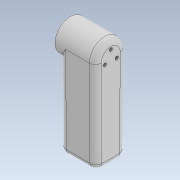
# Autodesk Inventor part: shank_link
Saved by Autodesk Inventor 2020 (Build 240168000, 168)
## iProperties
Created: 2020-12-22
Part Number: shank_link
Material: Generic
Document SubType Name: Modeling
Designer: DELL
Density: 1 g/cm^3
Appearance: Default
Author: DELL
Autodesk Inventor part; units mm, degrees
ref_plane "XY Plane" through (0, 0, 0) normal (0, 0, 1) x (1, 0, 0)
sketch "Sketch1" plane through (0, 0, 0) normal (1, 0, 0) x (0, 1, 0)
  line L0 (0, 0) -> (0, 25.2399) construction
  line L1 (0, 0) -> (0, -46.7601) construction
  line L2 (0, 0) -> (-156, 0) construction
  circle A0 centre (0, 0) radius 26
  line L3 (0, 0) -> (-13, 22.5167) construction
  line L4 (0, 0) -> (-13, -22.5167) construction
  line L5 (-0.1668, 25.9995) -> (-156, 25)
  line L6 (-0.1668, -25.9995) -> (-156, -25)
  line L7 (-156, 25) -> (-156, -25)
  circle A1 centre (0, 0) radius 11.5 construction
  circle A2 centre (11.5, 0) radius 1.65
  line L8 (0, 0) -> (26, 0) construction
  circle A3 centre (-5.75, 9.9593) radius 1.65
  circle A4 centre (-5.75, -9.9593) radius 1.65
  circle A5 centre (0, 0) radius 9.715 construction
  line L9 (0, 0) -> (5.75, 9.9593) construction
  line L10 (0, 0) -> (5.75, -9.9593) construction
  circle A6 centre (4.8575, 8.4134) radius 2
  circle A7 centre (4.8575, -8.4134) radius 2
  circle A8 centre (-9.715, 0) radius 2
  circle A9 centre (11.5, 0) radius 2.75
  circle A10 centre (-5.75, -9.9593) radius 2.75
  circle A11 centre (-5.75, 9.9593) radius 2.75
  circle A12 centre (0, 0) radius 156 construction
  arc A13 (-153.9817, 25.0129) -> (-153.9817, -25.0129) centre (0, 0) ccw
  line L11 (0, 0) -> (-0.1668, 25.9995) construction
  point P0 (-78, 0)
  dimension "d6" = 52
  dimension "d8" = 60
  dimension "d84" = 156
  dimension "d85" = 50
  dimension "d97" = 23
  dimension "d98" = 3.3
  dimension "d99" = 19.43
  dimension "d100" = 30
  dimension "d101" = 4
  dimension "d102" = 5.5
  dimension "d129" = 25.0129
  dimension "d130" = 153.9817
  dimension "d131" = 2.0183
  constraints: 24 end point, 18 point on circle, 14 centre point, 10 point on line, 7 coincident, 6 equal radius, 2 midpoint, 2 vertical, 1 horizontal, 1 perpendicular, 1 symmetric about line, 1 tangent, 3 other
  measures "d6" diameter of A0
  measures "d8" angle of L2 L3
  measures "d84" distance between parallel lines of L7 L1
  measures "d85" distance of L5.end L6.end
  measures "d97" diameter of A1
  measures "d98" diameter of A2
  measures "d99" diameter of A5
  measures "d100" angle of L0 L9
  measures "d101" diameter of A6
  measures "d102" diameter of A9
  measures "d129" distance from line of A12.end L2
  measures "d130" distance from line of L0 A12.end
  measures "d131" distance from line of L7 A12.end
ref_plane "Work Plane1" through (14.5, 0, 0) normal (1, 0, 0) x (0, 1, 0)
ref_plane "Work Plane2" through (20, 0, 0) normal (1, 0, 0) x (0, 1, 0)
extrude "Extrusion4" add sketch "Sketch1" along normal mid plane 70 contours A0 | A6 | A7 | A8 | A9 | A10 | A11
extrude "Extrusion6" cut sketch "Sketch1" against normal blind 40 from surface at 35 contours A9 | A10 | A11
extrude "Extrusion7" cut sketch "Sketch1" along normal blind 5 from surface at -35 contours A6 | A7 | A8
extrude "Extrusion9" add sketch "Sketch1" against normal blind 60 from surface at 35 contours A0 L6 A13 L5
sketch "Sketch6" plane through (0, 0, 0) normal (0, 1, 0) x (-1, 0, 0)
  circle A0 centre (-5, 0) radius 10
  line L0 (25, 25.0129) -> (25, 25.9995) projected
  line L1 (25, 25.9995) -> (25, -25.9995) projected
  line L2 (25, -25.9995) -> (25, -25.0129) projected
  line L3 (25, -25.0129) -> (25, 25.0129) projected
  line L4 (-35, -12.7093) -> (-35, -7.2093) projected
  line L5 (-35, 7.2093) -> (-35, 12.7093) projected
  line L6 (-35, -2.75) -> (-35, 2.75) projected
  line L7 (-35, 25.0129) -> (-35, 25.9995) projected
  line L8 (-35, -25.0129) -> (-35, 25.0129) projected
  line L9 (-35, -25.9995) -> (-35, -25.0129) projected
  line L10 (-35, -25.9995) -> (-35, 25.9995) projected
  line L11 (25, 0) -> (-35, 0)
  dimension "d123" = 20
  constraints: 3 midpoint, 2 end point, 1 centre point, 1 coincident
  measures "d123" diameter of A0
ref_plane "Work Plane4" through (0, -156, 0) normal (0, 1, 0) x (-1, 0, 0)
extrude "Extrusion11" cut sketch "Sketch6" along normal blind 60 from surface at -156
fillet "Fillet28" radius 10 6 edges at (35, 18.3257, -18.4436) (35, 18.3257, 18.4436) (35, -77.0742, -25.5062) (35, -77.0742, 25.5062) (-25, -77.0742, 25.5062) (-25, -77.0742, -25.5062)
fillet "Fillet29" radius 8 2 edges at (5, -153.9817, -25.0129) (5, -153.9817, 25.0129)
fillet "Fillet33" radius 2 3 edges at (4.9872, -155.6792, 10) (4.9875, -155.6792, -10) (15, -96, 0)
fillet "Fillet34" radius 3 3 edges at (-20.7828, -9.7659, -24.0962) (-21.2433, -10.5931, 23.7442) (-25, -26, 0)
fillet "Fillet35" radius 2 1 edges at (-35, -26, 0)
body "Solid1"
